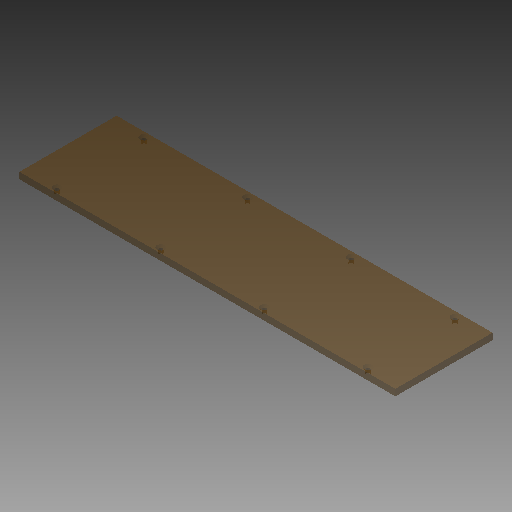
# Autodesk Inventor part: Tunneldecke
Saved by Autodesk Inventor 2018 (Build 220112000, 112)
## iProperties
Created: 2013-02-19
Part Number: Tunneldecke
Material: Polycarbonate, Clear
Document SubType Name: Modeling
Designer: Neef
Mass: 129.999 g
Surface Area: 473.738 cm^2
Volume: 108.332 cm^3
Density: 1.2 g/cm^3
Appearance: Polycarbonate - Smoked
Author: Neef
Autodesk Inventor part; units mm, degrees
ref_plane "YZ Plane" through (0, 0, 0) normal (1, 0, 0) x (0, 1, 0)
ref_plane "XZ Plane" through (0, 0, 0) normal (0, 1, 0) x (-1, 0, 0)
ref_plane "XY Plane" through (0, 0, 0) normal (0, 0, 1) x (1, 0, 0)
sketch "Skizze1" plane through (0, 0, 0) normal (0, 0, 1) x (1, 0, 0)
  line L0 (145, -37.5) -> (-145, -37.5)
  line L1 (-145, -37.5) -> (-145, 37.5)
  line L2 (-145, 37.5) -> (145, 37.5)
  line L3 (145, 37.5) -> (145, -37.5)
  line L4 (0, 52.5) -> (0, -52.5) projected
  line L5 (-203, 0) -> (203, 0) projected
  point P0 (0, 0)
  point P1 (0, -37.5)
  point P2 (-145, 0)
  dimension "d0" = 290
  dimension "d1" = 75
  constraints: 8 end point, 2 midpoint, 2 parallel, 2 point on line, 1 horizontal, 1 perpendicular
  measures "d0" distance of L0.start L0.end
  measures "d1" distance of L0.end L1.end
extrude "Extrusion1" add sketch "Skizze1" along normal blind 5
sketch "Skizze2" plane through (0, 0, 5) normal (0, 0, 1) x (1, 0, 0)
  line L0 (-145, -37.5) -> (-145, 37.5) projected
  line L1 (145, -37.5) -> (-145, -37.5) projected
  point P0 (0, 0)
  point P1 (-120, -33.5)
  dimension "d4" = 25
  dimension "d5" = 4
  measures "d4" distance from line of L0 point (-120, -33.5)
  measures "d5" distance from line of L1 point (-120, -33.5)
hole "Bohrung1" at (-120, -33.5, 5) direction (0, 0, -1) diameter 3.1 end through all countersink diameter 6.1 countersink angle 90
pattern_linear "Rechteckige Anordnung1" count 4 spacing 80 along (1, 0, 0) count 2 spacing 67 along (0, 1, 0) of "Bohrung1"
